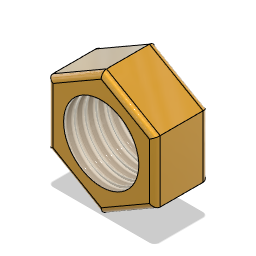
0.160.4837 - Ecrou H (Autodesk Fusion 360 design; units mm, degrees)
Autodesk Fusion 360 part; units mm, degrees
sketch "Sketch1" plane through (0, 0, 0) normal (0, 0, 1) x (1, 0, 0)
  circle A0 centre (0, 0) radius 8
  dimension "d1" = 16
  constraint coincident A0.centre origin
  measures "d1" diameter of A0
extrude "Extrude1" add sketch "Sketch1" along normal blind 55
sketch "Sketch2" plane through (0, 0, 0) normal (0, 0, -1) x (-1, 0, 0)
  circle A0 centre (0, 0) radius 8
  circle A1 centre (0, 0) radius 8
  line L0 (10, 5.7735) -> (0, 11.547)
  line L1 (0, 11.547) -> (-10, 5.7735)
  line L2 (-10, 5.7735) -> (-10, -5.7735)
  line L3 (-10, -5.7735) -> (0, -11.547)
  line L4 (0, -11.547) -> (10, -5.7735)
  line L5 (10, -5.7735) -> (10, 5.7735)
  constraint coincident A0.centre A1.centre
extrude "Extrude2" add sketch "Sketch2" along normal blind 10 contours A0 A1 | L0 L1 L2 L3 L4 L5
thread "Thread1" "ISO Metric profile 16.0 M16x2 6g" major diameter 15.822 minor diameter 13.534 pitch 2 angle 60 resizes the face on face at (7.9602, -0.7965, 18.3333)
fillet "Fillet1" radius 1 12 edges at (5, -8.6603, -10) (10, 0, -10) (5, 8.6603, -10) (-5, 8.6603, -10) (-10, 0, -10) (-5, -8.6603, -10) (5, -8.6603, 0) (10, 0, 0) (-5, -8.6603, 0) (-10, 0, 0) (-5, 8.6603, 0) (5, 8.6603, 0)
sketch "Sketch3" plane through (0, 0, 55) normal (0, 0, 1) x (1, 0, 0)
  circle A0 centre (0, 0) radius 7.911
  circle A1 centre (0, 0) radius 7.911
  circle A2 centre (0, 0) radius 7.911
extrude "Extrude3" cut sketch "Sketch3" against normal through all
thread "Thread2" "ISO Metric profile 16.0 M16x2 6H" major diameter 16.2505 minor diameter 14.0225 pitch 2 angle 60 resizes the face on face at (7.8717, 0.7877, -3.3333)
